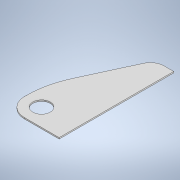
# Autodesk Inventor part: Beslag_stempel
Saved by Autodesk Inventor 2022 (Build 260153000, 153)
## iProperties
Created: 2022-04-09
Part Number: Beslag_stempel
Material: Generic
Document SubType Name: Sheet Metal
Designer: Patrick
Density: 1 g/cm^3
Sheet Metal Rule: Default_mm
Appearance: Default
Author: Patrick
Autodesk Inventor part; units mm, degrees
ref_plane "YZ Plane" through (0, 0, 0) normal (1, 0, 0) x (0, 1, 0)
ref_plane "XZ Plane" through (0, 0, 0) normal (0, 1, 0) x (-1, 0, 0)
ref_plane "XY Plane" through (0, 0, 0) normal (0, 0, 1) x (1, 0, 0)
sketch "Sketch1" plane through (0, 0, 0) normal (0, 1, 0) x (-1, 0, 0)
  line L0 (0, 0) -> (60, 0)
  line L1 (60, 0) -> (60, -45)
  line L2 (60, -45) -> (20.9424, -130)
  line L3 (20.9424, -130) -> (0, -130)
  line L4 (0, 0) -> (0, -130)
  circle A0 centre (40, -20) radius 10
  dimension "d0" = 45
  dimension "d1" = 40
  dimension "d2" = 20
  dimension "d3" = 20
  dimension "d4" = 130
  dimension "d5" = 20
  measures "d0" distance of L0.end L1.end
  measures "d1" distance from line of L4 A0.centre
  measures "d2" distance from line of A0.centre L0
  measures "d3" distance from line of L1 A0.centre
  measures "d4" distance of L0.start L3.end
  measures "d5" diameter of A0
extrude "Plate1" add sketch "Sketch1" along normal blind 1.5
fillet "Fillet1" radius 20.5 1 edges at (-60, 0.75, 0)
fillet "Fillet2" radius 103.25 1 edges at (-60, 0.75, -45)
fillet "Fillet3" radius 15.5 1 edges at (-20.9424, 0.75, -130)
equation "\"d6\" = Thickness"
equation "\"BendRadius\" = Thickness"
equation "\"BendReliefWidth\" = Thickness"
equation "\"BendReliefDepth\" = 0.5 * Thickness"
equation "\"CornerReliefSize\" = 4 * Thickness"
equation "\"MinimumRemnant\" = 2 * Thickness"
equation "\"TransitionRadius\" = BendRadius"
equation "\"JacobiRadiusSize\" = BendRadius"
equation "\"GapSize\" = Thickness"
equation "\"Thickness\" = 1.5"
body "Solid1"
